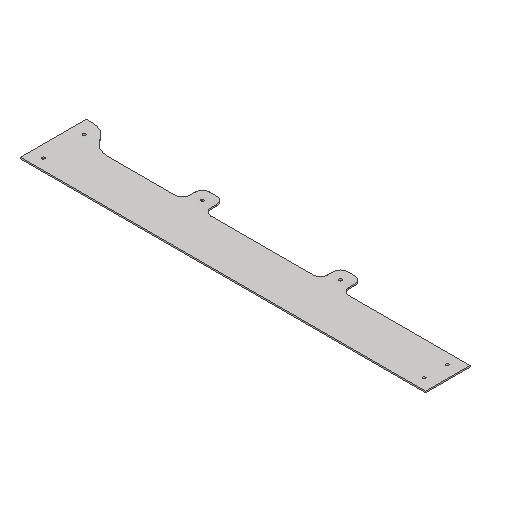
# Autodesk Inventor part: LC_ALU_2mm_Right_Plate
Saved by Autodesk Inventor 2026.1 (Build 301233000, 233)
## iProperties
Created: 2016-06-26
Part Number: LC_ALU_2mm_Right_Plate
Material: Ogólny
Document SubType Name: Modeling
Designer: Andrzej
Density: 1 g/cm^3
Appearance: Obrobione — aluminium
Mass: 73.3932 g
Surface Area: 762.113 cm^2
Volume: 73.3932 cm^3
Author: Andrzej
Autodesk Inventor part; units mm, degrees
ref_plane "YZ Plane" through (0, 0, 0) normal (1, 0, 0) x (0, 1, 0)
ref_plane "XZ Plane" through (0, 0, 0) normal (0, 1, 0) x (-1, 0, 0)
ref_plane "XY Plane" through (0, 0, 0) normal (0, 0, 1) x (1, 0, 0)
sketch "Szkic1" plane through (0, 0, 0) normal (0, 0, 1) x (1, 0, 0)
  line L0 (-98.62, 58.242) -> (467.38, 58.242)
  line L1 (467.38, 58.242) -> (467.38, -3.758)
  line L2 (467.38, -3.758) -> (-98.62, -3.758)
  line L3 (-98.62, -3.758) -> (-98.62, 58.242)
  line L4 (65.48, 58.242) -> (95.48, 58.242)
  line L5 (95.48, 58.242) -> (95.48, 86.242)
  line L6 (95.48, 86.242) -> (65.48, 86.242)
  line L7 (65.48, 86.242) -> (65.48, 58.242)
  line L8 (258.28, 58.242) -> (288.28, 58.242)
  line L9 (288.28, 58.242) -> (288.28, 86.242)
  line L10 (288.28, 86.242) -> (258.28, 86.242)
  line L11 (258.28, 86.242) -> (258.28, 58.242)
  line L12 (-98.62, 58.242) -> (-68.62, 58.242)
  line L13 (-68.62, 58.242) -> (-68.62, 88.242)
  line L14 (-68.62, 88.242) -> (-98.62, 88.242)
  line L15 (-98.62, 88.242) -> (-98.62, 58.242)
  point P0 (0, 0)
  point P1 (80.48, 71.242)
  point P2 (273.28, 71.242)
  point P3 (-81.62, 68.242)
  point P4 (450.38, 43.242)
  point P5 (-81.62, 11.242)
  point P6 (450.38, 11.242)
  dimension "d0" = 566
  dimension "d1" = 62
  dimension "d2" = 30
  dimension "d3" = 28
  dimension "d4" = 30
  dimension "d5" = 28
  dimension "d6" = 164.1
  dimension "d7" = 356.9
  dimension "d11" = 15
  dimension "d12" = 15
  dimension "d13" = 15
  dimension "d14" = 15
  dimension "d16" = 15
  dimension "d17" = 17
  dimension "d18" = 17
  dimension "d26" = 17
  dimension "d27" = 15
  dimension "d28" = 17
  dimension "d29" = 15
  dimension "d30" = 30
  dimension "d31" = 30
  dimension "d33" = 20
  constraints: 32 end point, 8 parallel, 4 horizontal, 4 perpendicular, 2 point on line
  measures "d0" distance of L1.end L2.end
  measures "d1" distance of L2.end L0.start
  measures "d2" distance of L6.end L5.end
  measures "d3" distance of L5.end L4.end
  measures "d4" distance of L10.end L9.end
  measures "d5" distance of L9.end L8.end
  measures "d6" distance between parallel lines of L3 L7
  measures "d7" distance between parallel lines of L3 L11
  measures "d11" distance from line of L6 point (80.48, 71.242)
  measures "d12" distance from line of L10 point (273.28, 71.242)
  measures "d13" distance from line of L7 point (80.48, 71.242)
  measures "d14" distance from line of L11 point (273.28, 71.242)
  measures "d16" distance from line of L0 point (450.38, 43.242)
  measures "d17" distance from line of L3 point (-81.62, 68.242)
  measures "d18" distance from line of L1 point (450.38, 43.242)
  measures "d26" distance from line of L3 point (-81.62, 11.242)
  measures "d27" distance from line of L2 point (-81.62, 11.242)
  measures "d28" distance from line of L1 point (450.38, 11.242)
  measures "d29" distance from line of L2 point (450.38, 11.242)
  measures "d30" distance of L14.end L13.end
  measures "d31" distance of L13.end L12.end
  measures "d33" distance from line of L14 point (-81.62, 68.242)
extrude "Wyciągnięcie proste1" add sketch "Szkic1" along normal blind 2
fillet "Zaokrąglenie1" radius 10 8 edges at (258.28, 58.242, 1) (258.28, 86.242, 1) (288.28, 86.242, 1) (288.28, 58.242, 1) (95.48, 58.242, 1) (95.48, 86.242, 1) (65.48, 86.242, 1) (65.48, 58.242, 1)
hole "Otwór1" at (80.48, 71.242, 0) at (273.28, 71.242, 0) at (-81.62, 68.242, 0) at (450.38, 43.242, 0) at (-81.62, 11.242, 0) at (450.38, 11.242, 0) direction (0, 0, 1) diameter 4 end through all
fillet "Zaokrąglenie2" radius 30 2 edges at (-68.62, 58.242, 1) (-68.62, 88.242, 1)
equation "\"d3\" = d5"
equation "\"d12\" = d11"
equation "\"d13\" = 0.5 * d2"
equation "\"d14\" = 0.5 * d4"
equation "\"d16\" = d15"
equation "\"d27\" = d15"
equation "\"d29\" = d16"
equation "\"d15\" = 15"
